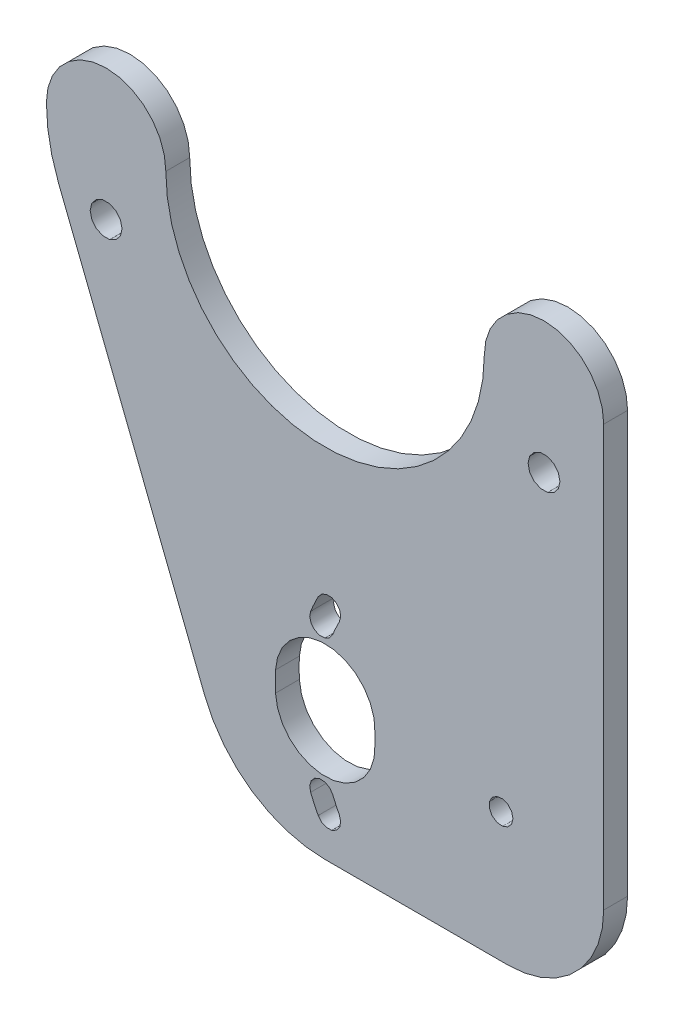
# Autodesk Inventor part: motor plate
Saved by Autodesk Inventor 2015 (Build 190159000, 159)
## iProperties
Created: 2015-08-29
Part Number: motor plate
Material: Generic
Description: insert part description/title
Document SubType Name: Modeling
Designer: francis
Density: 1 g/cm^3
Appearance: Default
Part Category: insert part category here and press enter to fill value
Author: francis
Autodesk Inventor part; units mm, degrees
ref_plane "YZ Plane" through (0, 0, 0) normal (1, 0, 0) x (0, 1, 0)
ref_plane "XZ Plane" through (0, 0, 0) normal (0, 1, 0) x (-1, 0, 0)
ref_plane "XY Plane" through (0, 0, 0) normal (0, 0, 1) x (1, 0, 0)
sketch "Sketch1" plane through (0, 0, 0) normal (0, 0, 1) x (1, 0, 0)
  line L0 (-15, 13.1624) -> (0, 13.1624) construction
  line L1 (-15, -13.1624) -> (-15, 13.1624) construction
  line L2 (0, -13.1624) -> (-15, -13.1624) construction
  line L3 (0, 13.1624) -> (0, -13.1624) construction
  circle A0 centre (20, -58.85) radius 1.2295 construction
  circle A1 centre (20, -38.35) radius 1.2295 construction
  circle A2 centre (42.1, -48.6) radius 1.2295 construction
  circle A3 centre (20, -48.6) radius 6 construction
  circle A4 centre (20, 0) radius 4 construction
  line L4 (40, 13.1624) -> (55, 13.1624) construction
  line L5 (40, -13.1624) -> (40, 13.1624) construction
  line L6 (55, -13.1624) -> (40, -13.1624) construction
  line L7 (55, 13.1624) -> (55, -13.1624) construction
  arc A5 (0, 0) -> (-15, 0) centre (-7.5, 0) ccw
  arc A6 (55, 0) -> (40, 0) centre (47.5, 0) ccw
  arc A7 (0, 0) -> (40, 0) centre (20, 0) ccw
  line L8 (53.51, -48.6) -> (3.95, -48.6) construction
  line L9 (20, -64.85) -> (43, -64.85)
  line L10 (55, 0) -> (55, -52.85)
  arc A8 (43, -64.85) -> (55, -52.85) centre (43, -52.85) ccw
  line L11 (4.8831, -54.5617) -> (-13.4793, -8.001)
  arc A9 (4.8831, -54.5617) -> (20, -64.85) centre (20, -48.6) ccw
  arc A10 (-15, 0) -> (-13.4793, -8.001) centre (6.8084, 0) ccw
  circle A11 centre (42.1, -48.6) radius 1.5
  arc A12 (19.1333, -36.7114) -> (18.1846, -38.7583) centre (42.1, -48.6) ccw
  arc A13 (21.7975, -38.0905) -> (20.9588, -39.9) centre (42.1, -48.6) ccw
  arc A14 (20.9609, -57.3051) -> (21.8001, -59.1144) centre (42.1, -48.6) ccw construction
  arc A15 (18.1869, -58.4474) -> (19.1362, -60.4941) centre (42.1, -48.6) ccw
  arc A16 (19.1362, -60.4941) -> (21.8001, -59.1144) centre (20.4681, -59.8042) ccw
  arc A17 (20.9609, -57.3051) -> (18.1869, -58.4474) centre (19.5739, -57.8763) ccw
  arc A18 (18.1846, -38.7583) -> (20.9588, -39.9) centre (19.5717, -39.3292) ccw
  arc A19 (21.7975, -38.0905) -> (19.1333, -36.7114) centre (20.4654, -37.401) ccw
  arc A20 (19.5739, -57.8763) -> (20.4681, -59.8042) centre (42.1, -48.6) ccw construction
  arc A21 (20.4654, -37.401) -> (19.5717, -39.3292) centre (42.1, -48.6) ccw construction
  arc A22 (20.9609, -57.3051) -> (21.8001, -59.1144) centre (42.1, -48.6) ccw
  arc A23 (13.7784, -47.3325) -> (13.7784, -49.8675) centre (39.8451, -48.6) ccw
  arc A24 (26.2637, -47.9396) -> (26.2637, -49.2604) centre (39.8451, -48.6) ccw
  arc A25 (13.7784, -49.8675) -> (26.2637, -49.2604) centre (20.021, -49.564) ccw
  arc A26 (26.2637, -47.9396) -> (13.7784, -47.3325) centre (20.021, -47.636) ccw
  arc A27 (20.021, -47.636) -> (20.021, -49.564) centre (42.1, -48.6) ccw construction
  circle A28 centre (-7.5, -9) radius 1.7295
  circle A29 centre (47.5, -9) radius 1.7295
  circle A30 centre (47.5, -9) radius 2
  circle A31 centre (-7.5, -9) radius 2
  circle A32 centre (-10.5, 0) radius 2.067
  circle A33 centre (44.5, 0) radius 2.067
extrude "Extrusion1" add sketch "Sketch1" along normal blind 3 contours A7 A6 L10 A8 L9 A9 L11 A10 A5 | A32 | A33
body "Solid1"
